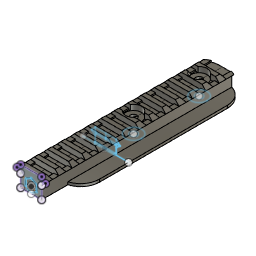
2023_01_22_Atomstack ProPlus PicaTinnyHolder v2 (Autodesk Fusion 360 design; units mm, degrees)
Autodesk Fusion 360 part; units mm, degrees
note: some values were not read from the file. Set by a fixed rule: which face or edge a step refers to.
sketch "Esquisse1" plane through (0, 0, 0) normal (0, 0, 1) x (1, 0, 0)
  line L0 (0, 0) -> (34, 0)
  line L1 (34, 0) -> (34, 88)
  line L2 (34, 88) -> (0, 88)
  line L3 (0, 88) -> (0, 0)
  line L4 (0, 0) -> (34, 0)
  line L5 (34, 0) -> (34, -35.2222)
  line L6 (34, -35.2222) -> (0, -35.2222)
  line L7 (0, -35.2222) -> (0, 0)
  dimension "d1" = 34
  dimension "d2" = 88
  constraint horizontal L0
  constraint vertical L1
  constraint horizontal L2
  constraint vertical L3
  constraint coincident L0.start L3.end
  constraint horizontal L4
  constraint vertical L5
  constraint horizontal L6
  constraint vertical L7
  measures "d1" distance of L0.start L0.end
  measures "d2" distance of L0.start L2.end
extrude "Extrusion1" add sketch "Esquisse1" along normal blind 1.95 contours L0 L1 L2 L3 L4 makes body 1
sketch "Esquisse3" plane through (0, 0, 0) normal (0, 1, 0) x (1, 0, 0)
  line L0 (16.9722, -9.3997) -> (27.5722, -9.3997)
  line L1 (6.3722, -9.3997) -> (9.1372, -6.8513)
  line L2 (16.9722, -8.3997) -> (24.0237, -8.3997)
  line L3 (9.1372, -12.3997) -> (9.1372, -3.0797)
  line L4 (27.5722, -9.3997) -> (24.8072, -6.8513)
  line L5 (9.9207, -8.3997) -> (9.9207, -9.3997)
  line L6 (24.0237, -8.3997) -> (24.0237, -9.3997)
  line L7 (24.8072, -12.3997) -> (27.5722, -9.3997)
  line L8 (6.3722, -9.3997) -> (9.1372, -12.3997)
  line L9 (24.8072, -12.3997) -> (9.1372, -12.3997)
  line L10 (24.8072, -3.0797) -> (24.8072, -12.3997)
  line L11 (16.9722, -12.3997) -> (16.9722, -9.3997)
  line L12 (9.1372, -3.0797) -> (24.8072, -3.0797)
  line L13 (16.9722, -9.3997) -> (16.9722, -8.3997)
  line L14 (16.9722, -8.3997) -> (9.9207, -8.3997)
  line L15 (16.9722, -9.3997) -> (6.3722, -9.3997)
sketch "Esquisse4" plane through (0, 0, 0) normal (0, 1, 0) x (1, 0, 0)
  line L0 (0, -2) -> (34, -2)
  line L1 (23.2949, -1.4559) -> (8.7051, -1.4559)
  line L2 (8.7051, -1.4559) -> (8.7051, -2.5441)
  line L3 (8.7051, -2.5441) -> (23.2949, -2.5441)
  line L4 (23.2949, -2.5441) -> (23.2949, -1.4559)
  line L5 (23.2949, -1.4559) -> (8.7051, -2.5441) construction
  line L6 (8.7051, -1.4559) -> (23.2949, -2.5441) construction
  point P0 (16, -2)
  constraint horizontal L0
  constraint horizontal L1
  constraint perpendicular L1 L2
  constraint parallel L1 L3
  constraint parallel L2 L4
  constraint coincident L5 P0
  constraint coincident L6 P0
  constraint coincident L0 P0
extrude "Extrusion2" add sketch "Esquisse4" along normal blind 88 separate body makes body 2
extrude "Extrusion3" add 1 faces at (13.5684, 29.3333, 2.5441) along direction (0, 0, 1) blind 1.5 on bodies 2 bodies 2
extrude "Extrusion4" add sketch "Esquisse3" along normal blind 5.25 separate body contours L0 L2 L3 L5 L6 L10 L12 L14 L15 | L0 L4 L10 | L1 L3 L15 makes body 3
extrude "Extrusion5" add sketch "Esquisse3" 1 faces at (16.9722, 0, 4.853) along normal blind 4.75 separate body contours L0 L2 L6 L13 | L0 L9 L10 L11 | L5 L13 L14 L15 | L3 L9 L11 L15 | L0 L7 L10 | L3 L8 L15 on bodies 3 makes body 4
move_body "Déplacer9" bodies 4 to x (1, 0, 0) y (0, 1, 0) z (0, 0, 1) at (0, -5, 0)
move_body "Déplacer10" bodies 4 to x (1, 0, 0) y (0, 1, 0) z (0, 0, 1) at (0, 0.25, 0)
combine "Combiner1" operation add target body 4 tool bodies 3
draft "Dépouille1" angle 20 neutral plane through (16.9722, 0, 8.3997) pull (0, 0, 1) 1 faces at (19.3227, 0, 11.3997) on bodies 4
draft "Dépouille2" angle 15 neutral plane through (16.9722, -4.75, 12.3997) pull (0, 0, 1) 1 faces at (19.3227, -1.0919, 11.3997) on bodies 4
pattern_linear "Réseau R1" count 6 spacing 10 along (0, -1, 0) of bodies 4 makes body 5 at (14.3605, -14.75, 10.5502) makes body 6 at (14.3605, -24.75, 10.5502) makes body 7 at (14.3605, -34.75, 10.5502) makes body 8 at (14.3605, -44.75, 10.5502) makes body 9 at (14.3605, -54.75, 10.5502)
pattern_linear "Réseau R2" count 10 spacing 10 along (0, 1, 0) of bodies 4 makes body 10 at (14.3605, 5.25, 10.5502) makes body 11 at (14.3605, 15.25, 10.5502) makes body 12 at (14.3605, 25.25, 10.5502) makes body 13 at (14.3605, 35.25, 10.5502) makes body 14 at (14.3605, 45.25, 10.5502) makes body 15 at (14.3605, 55.25, 10.5502) makes body 16 at (14.3605, 65.25, 10.5502) makes body 17 at (14.3605, 75.25, 10.5502) makes body 18 at (14.3605, 85.25, 10.5502)
combine "Combiner2" operation add target body 9 tool bodies 8 7 5 4 6 10 11 12 13 14 15 18 17 16
move_body "Déplacer1" bodies 9 to x (1, 0, 0) y (0, 1, 0) z (0, 0, 1) at (-1, 0, 1)
extrude "Extrusion6" add 1 faces at (23.2949, 29.3333, 3.1814) along direction (1, 0, 0) blind 0.512 on bodies 2 bodies 2 1
extrude "Extrusion7" add 1 faces at (8.7051, 29.3333, 2.648) along direction (-1, 0, 0) blind 0.568 on bodies 2 bodies 2
move_body "Déplacer2" bodies 9 to x (1, 0, 0) y (0, 1, 0) z (0, 0, 1) at (0, 0, 1.5)
extrude "Extrusion8" add 1 faces at (13.3605, -4.75, 5.5797) along direction (0, 0, -1) blind 4.08 on bodies 9 bodies 9 2
extrude "Extrusion10" add 1 faces at (13.3605, -36.5, 1.4997) along direction (0, 0, -1) blind 1.5 on bodies 9 bodies 9
sketch "Esquisse6" plane through (0, -54.75, 0) normal (0, -1, 0) x (1, 0, 0)
  line L0 (19.8929, 7.7966) -> (15.9337, 10.061)
  line L1 (15.9337, 10.061) -> (11.993, 7.7645)
  line L2 (11.993, 7.7645) -> (12.0115, 3.2034)
  line L3 (12.0115, 3.2034) -> (15.9708, 0.939)
  line L4 (15.9708, 0.939) -> (19.9115, 3.2355)
  line L5 (19.9115, 3.2355) -> (19.8929, 7.7966)
  line L6 (8.1372, 9.3513) -> (23.8072, -0.0003) construction
  line L7 (23.8072, 9.3513) -> (8.1372, -0.0003) construction
  line L8 (15.9722, 4.6755) -> (15.9722, -0.0003) construction
  line L9 (26.5722, 11.8997) -> (23.8072, 14.8997)
  line L10 (23.8072, 14.8997) -> (8.1372, 14.8997)
  line L11 (8.1372, 14.8997) -> (5.3722, 11.8997)
  line L12 (5.3722, 11.8997) -> (8.1372, 9.3513)
  line L13 (8.1372, 9.3513) -> (8.1372, -0.0003)
  line L14 (8.1372, -0.0003) -> (23.8072, -0.0003)
  line L15 (23.8072, -0.0003) -> (23.8072, 9.3513)
  line L16 (23.8072, 9.3513) -> (26.5722, 11.8997)
  line L17 (11.6923, 7.9364) -> (11.7122, 3.029)
  line L18 (11.7122, 3.029) -> (15.9722, 0.5926)
  line L19 (15.9722, 0.5926) -> (20.2122, 3.0636)
  line L20 (20.2122, 3.0636) -> (20.1922, 7.971)
  line L21 (20.1922, 7.971) -> (15.9323, 10.4074)
  line L22 (15.9323, 10.4074) -> (11.6923, 7.9364)
  point P0 (15.9522, 5.5)
  point P1 (15.9722, 4.6755)
  dimension "d35" = 3.95
  dimension "d77" = 0.3
  constraint midpoint L7 P1
  constraint coincident P1 L8.start
  measures "d35" distance of P0 L5
extrude "Extrusion12" add 1 faces at (13.3605, 90.4167, 1.4997) along direction (0, 0, -1) blind 1.5 on bodies 9 bodies 9
extrude "Extrusion11" cut sketch "Esquisse6" against normal blind 158 contours L0 L1 L2 L3 L4 L5 bodies 9
copy_body "Copier/Coller des corps1" bodies 9 makes body 19
extrude "Extrusion20" cut 1 faces at (22.5086, 95.25, 4.1955) along direction (0, -1, 0) blind 7.25 on bodies 19 bodies 9 19
extrude "Extrusion21" cut 1 faces at (18.3227, 85.25, 13.8997) along direction (0, 1, 0) blind 14 on bodies 19 bodies 9 19
combine "Combiner3" operation add target body 9 tool bodies 19
extrude "Extrusion22" cut sketch "Esquisse6" against normal blind 191 contours L17 L18 L19 L20 L21 L22 bodies 9
fillet "Congé4" radius 10 4 edges at (0, 88, 0.975) (34, 88, 0.975) (0, 0, 0.975) (34, 0, 0.975) on bodies 9
sketch "Esquisse9" plane through (0, 0, 0) normal (0, 0, 1) x (1, 0, 0)
  circle A0 centre (15.4326, 71.3659) radius 6
  circle A1 centre (15.4326, 71.3659) radius 2.5
  circle A2 centre (15.4326, 22.3659) radius 2.5
  circle A3 centre (15.4326, 22.3659) radius 6
  dimension "d84" = 5
  dimension "d85" = 12
  dimension "d96" = 5
  dimension "d97" = 12
  constraint concentric A0 A1
  constraint concentric A2 A3
  measures "d84" diameter of A1
  measures "d85" diameter of A0
  measures "d96" diameter of A2
  measures "d97" diameter of A3
extrude "Extrusion23" cut sketch "Esquisse9" along normal blind 28 contours A0 | A1 | A2 | A3 bodies 9
extrude "Extrusion24" add sketch "Esquisse9" along normal blind 10.9 bodies 9
extrude "Extrusion25" cut sketch "Esquisse6" against normal blind 165 contours L0 L1 L2 L3 L4 L5 | L17 L18 L19 L20 L21 L22 bodies 9
extrude "Extrusion26" add sketch "Esquisse1" along normal blind 1.95 bodies 9
fillet "Congé5" radius 14 4 edges at (34, -35.2222, 0.975) (34, 88, 0.975) (0, 88, 0.975) (0, -35.2222, 0.975) on bodies 9
equation "d35 = ( 7.9 / 2 ) * 1 mm"
